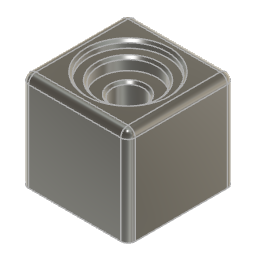
_Magnet Gluing Adapter.a96ae204-5c2f-496e-8506-899d32d27325 (Autodesk Fusion 360 design; units mm, degrees)
Autodesk Fusion 360 part; units mm, degrees
note: some values were not read from the file. Set by a fixed rule: which sketch regions a step uses.
sketch "Sketch1" plane through (0, 0, 0) normal (0, 0, 1) x (1, 0, 0)
  line L0 (0, 0) -> (-44, 0)
  line L1 (-44, 0) -> (-44, 44)
  line L2 (-44, 44) -> (0, 44)
  line L3 (0, 44) -> (0, 0)
  dimension "d1" = 44
  dimension "d2" = 44
  constraint horizontal L0
  constraint vertical L1
  constraint horizontal L2
  constraint vertical L3
  constraint coincident L0.start L3.end
  measures "d1" distance of L0.start L0.end
  measures "d2" distance of L0.start L2.end
extrude "Extrude1" add sketch "Sketch1" along normal blind 40
sketch "Sketch2" plane through (0, 0, 40) normal (0, 0, 1) x (-1, 0, 0)
  line L0 (0, -44) -> (44, -44)
  line L1 (44, -44) -> (44, 0)
  line L2 (44, 0) -> (0, 0)
  line L3 (0, 0) -> (0, -44)
  line L4 (44, -44) -> (0, 0)
  line L5 (0, -44) -> (44, 0)
  circle A0 centre (22, -22) radius 16.25
  dimension "d5" = 32.5
  constraint coincident L0.end L1.start
  constraint coincident L2.end L3.start
  constraint coincident L0.start L3.end
  constraint coincident L1.end L2.start
  constraint midpoint L5 A0.centre
  measures "d5" diameter of A0
extrude "Extrude2" cut sketch "Sketch2" against normal blind 3 contours L4 L5 A0 | L4 L5 A0 | L4 L5 A0 | L4 L5 A0
sketch "Sketch3" plane through (0, 0, 37) normal (0, 0, 1) x (-1, 0, 0)
  circle A0 centre (22, -22) radius 16.25
  circle A1 centre (22, -22) radius 12
  dimension "d8" = 24
  constraint concentric A0 A1
  measures "d8" diameter of A1
extrude "Extrude3" cut sketch "Sketch3" against normal blind 5 contours A1
sketch "Sketch4" plane through (0, 0, 32) normal (0, 0, 1) x (-1, 0, 0)
  circle A0 centre (22, -22) radius 12
  circle A1 centre (22, -22) radius 6.45
  dimension "d11" = 12.9
  constraint concentric A0 A1
  measures "d11" diameter of A1
extrude "Extrude4" cut sketch "Sketch4" against normal blind 50 contours A1
fillet "Fillet1" radius 3 8 edges at (-22, 44, 40) (-44, 22, 40) (-22, 0, 40) (0, 22, 40) (0, 0, 20) (-44, 0, 20) (0, 44, 20) (-44, 44, 20)
chamfer "Chamfer1" distance 1 angle 45 3 edges at (-10.8121, 17.6606, 37) (-15.9865, 19.6676, 32) (-6.8497, 16.1237, 40)
